Autodesk Fusion 360 part; units mm, degrees
note: some values were not read from the file. Chosen so that the rebuilt part matches the saved one: which face or edge a step refers to. Set by a fixed rule: which sketch regions a step uses; the direction of a hole.
(part 3 of 4)
sketch "Sketch120" plane through (0, -75, 0) normal (0, 1, 0) x (-1, 0, 0)
  line L0 (-100, 0) -> (-100, -5)
  line L1 (-100, -5) -> (-90, -5)
  line L2 (-90, -5) -> (-90, 3.5)
  line L3 (-90, 3.5) -> (-100, 3.5)
  line L4 (-100, 3.5) -> (-100, 50)
  line L5 (-100, 50) -> (-162.3, 50)
  line L6 (-162.3, 50) -> (-162.3, 3.5)
  line L7 (-162.3, 3.5) -> (-172.3, 3.5)
  line L8 (-172.3, 3.5) -> (-172.3, -5)
  line L9 (-172.3, -5) -> (-162.3, -5)
  line L10 (-162.3, -5) -> (-162.3, 0)
  line L11 (-162.3, 0) -> (-100, 0)
  line L12 (-162.3, 45) -> (-152.3, 45)
  line L13 (-152.3, 45) -> (-152.3, 42)
  line L14 (-152.3, 42) -> (-162.3, 42)
  line L15 (-162.3, 42) -> (-162.3, 45)
  line L16 (-100, 45) -> (-110, 45)
  line L17 (-110, 45) -> (-110, 42)
  line L18 (-110, 42) -> (-100, 42)
  line L19 (-100, 42) -> (-100, 45)
  line L20 (-162.3, 50) -> (-100, 50)
  dimension "d903" = 10
  dimension "d904" = 3
  dimension "d905" = 5
  dimension "d906" = 10
  dimension "d907" = 3
  dimension "d908" = 5
  constraint horizontal L12
  constraint vertical L13
  constraint horizontal L14
  constraint vertical L15
  constraint coincident L6 L12.start
  constraint horizontal L16
  constraint vertical L17
  constraint horizontal L18
  constraint vertical L19
  constraint coincident L4 L16.start
  measures "d903" distance of L12.start L12.end
  measures "d904" distance of L12.start L14.end
  measures "d905" distance of L5 L12
  measures "d906" distance of L16.start L16.end
  measures "d907" distance of L16.start L18.end
  measures "d908" distance of L16 L20
extrude "Extrude160" cut sketch "Sketch120" against normal blind 10 contours L4 L16 L17 L18 L19 | L6 L12 L13 L14 L15 bodies 7
extrude "Extrude161" add sketch "Sketch119" along normal blind 5 contours L4 L10 L14 L15 L16 L17 bodies 7
sketch "Sketch121" plane through (0, 0, 0) normal (0, 0, 1) x (1, 0, 0)
  line L0 (90, -100) -> (172.3, -100)
  line L1 (172.3, -100) -> (172.3, -145)
  line L2 (172.3, -145) -> (90, -145)
  line L3 (90, -145) -> (90, -100)
  line L4 (100, -100) -> (110, -100)
  line L5 (110, -100) -> (110, -110)
  line L6 (110, -110) -> (100, -110)
  line L7 (100, -110) -> (100, -100)
  line L8 (100, -145) -> (110, -145)
  line L9 (110, -145) -> (110, -135)
  line L10 (110, -135) -> (100, -135)
  line L11 (100, -135) -> (100, -145)
  line L12 (152.3, -100) -> (162.3, -100)
  line L13 (162.3, -100) -> (162.3, -110)
  line L14 (162.3, -110) -> (152.3, -110)
  line L15 (152.3, -110) -> (152.3, -100)
  line L16 (152.3, -145) -> (162.3, -145)
  line L17 (162.3, -145) -> (162.3, -135)
  line L18 (162.3, -135) -> (152.3, -135)
  line L19 (152.3, -135) -> (152.3, -145)
  circle A0 centre (105, -105) radius 2.5
  circle A1 centre (105, -140) radius 2.5
  circle A2 centre (157.3, -140) radius 2.5
  circle A3 centre (157.3, -105) radius 2.5
  line L20 (110, -100) -> (152.3, -100)
  line L21 (152.3, -100) -> (152.3, -110)
  line L22 (152.3, -110) -> (110, -110)
  line L23 (110, -110) -> (110, -100)
  line L24 (110, -135) -> (152.3, -135)
  line L25 (152.3, -135) -> (152.3, -145)
  line L26 (152.3, -145) -> (110, -145)
  line L27 (110, -145) -> (110, -135)
  circle A4 centre (131.15, -122.5) radius 8.5
  line L28 (172.3, -100) -> (90, -100)
  line L29 (90, -100) -> (90, -97)
  line L30 (90, -97) -> (172.3, -97)
  line L31 (172.3, -97) -> (172.3, -100)
  line L32 (90, -145) -> (172.3, -145)
  line L33 (172.3, -145) -> (172.3, -148)
  line L34 (172.3, -148) -> (90, -148)
  line L35 (90, -148) -> (90, -145)
  circle A5 centre (152.3, -110) radius 1
  circle A6 centre (152.3, -100) radius 1
  circle A7 centre (110, -110) radius 1
  circle A8 centre (110, -100) radius 1
  circle A9 centre (110, -135) radius 1
  circle A10 centre (110, -145) radius 1
  circle A11 centre (152.3, -145) radius 1
  circle A12 centre (152.3, -135) radius 1
  dimension "d913" = 82.3
  dimension "d914" = 45
  dimension "d915" = 10
  dimension "d916" = 10
  dimension "d917" = 10
  dimension "d918" = 10
  dimension "d919" = 10
  dimension "d920" = 5
  dimension "d921" = 5
  dimension "d922" = 5
  dimension "d923" = 5
  dimension "d930" = 17
  dimension "d1117" = 3
  dimension "d1118" = 3
  dimension "d1119" = 2
  dimension "d1120" = 2
  dimension "d1121" = 2
  dimension "d1122" = 2
  dimension "d1123" = 2
  dimension "d1124" = 2
  dimension "d1125" = 2
  dimension "d1126" = 2
  constraint horizontal L0
  constraint vertical L1
  constraint horizontal L2
  constraint vertical L3
  constraint horizontal L4
  constraint vertical L5
  constraint horizontal L6
  constraint vertical L7
  constraint coincident L0 L4.start
  constraint horizontal L8
  constraint vertical L9
  constraint horizontal L10
  constraint vertical L11
  constraint coincident L2 L8.start
  constraint horizontal L12
  constraint vertical L13
  constraint horizontal L14
  constraint vertical L15
  constraint coincident L0 L12.start
  constraint horizontal L16
  constraint vertical L17
  constraint horizontal L18
  constraint vertical L19
  constraint coincident L2 L16.start
  constraint horizontal L20
  constraint vertical L21
  constraint horizontal L22
  constraint vertical L23
  constraint horizontal L24
  constraint vertical L25
  constraint horizontal L26
  constraint vertical L27
  constraint horizontal L28
  constraint vertical L29
  constraint horizontal L30
  constraint vertical L31
  constraint horizontal L32
  constraint vertical L33
  constraint horizontal L34
  constraint vertical L35
  constraint coincident L14.end L15.start
  constraint coincident L12.start L15.end
  constraint coincident L5.end L6.start
  constraint coincident L4.end L5.start
  constraint coincident L9.end L10.start
  constraint coincident L8.end L9.start
  constraint coincident L16.start L19.end
  constraint coincident L18.end L19.start
  measures "d913" distance of L0.start L0.end
  measures "d914" distance of L0.start L2.end
  measures "d915" distance of L12.start L12.end
  measures "d916" distance of L16.start L16.end
  measures "d917" distance of L16.start L18.end
  measures "d918" distance of L1 L13
  measures "d919" distance of L1 L17
  measures "d920" diameter of A0
  measures "d921" diameter of A1
  measures "d922" diameter of A2
  measures "d923" diameter of A3
  measures "d930" diameter of A4
  measures "d1117" distance of L2.end L34.end
  measures "d1118" distance of L0.end L30.end
  measures "d1119" diameter of A5
  measures "d1120" diameter of A6
  measures "d1121" diameter of A7
  measures "d1122" diameter of A8
  measures "d1123" diameter of A9
  measures "d1124" diameter of A10
  measures "d1125" diameter of A11
  measures "d1126" diameter of A12
extrude "Extrude162" add sketch "Sketch121" along normal blind 10 separate body contours L0 L4 L12 L20 L28 L29 L30 L31 A6 A8 | L0 L1 L2 L3 L6 L7 L10 L11 L13 L14 L17 L18 L22 L24 L28 L32 A5 A7 A9 A12 | L0 L4 L5 L6 L7 L23 L28 A7 A8 | L2 L8 L16 L26 L32 L33 L34 L35 A10 A11 | L2 L8 L9 L10 L11 L27 L32 A9 A10 | L0 L12 L13 L14 L15 L21 L28 A5 A6 | L2 L16 L17 L18 L19 L25 L32 A11 A12 | A4 makes body 9
extrude "Extrude163" add sketch "Sketch121" along normal blind 5 contours L0 L4 L20 L28 A8 | L0 L4 L5 L23 L28 A8 | L0 L5 L20 L23 L28 A8 | L0 L5 L15 L20 L21 L22 L23 L28 A5 A6 A7 A8 | L5 L6 L23 A7 | L6 L22 A7 | L2 L8 L9 L27 L32 A10 | L2 L8 L26 L32 A10 | L0 L12 L20 L28 A6 | L0 L15 L20 L21 L28 A6 | L5 L22 L23 A7 | L2 L9 L26 L27 L32 A10 | L2 L9 L19 L24 L25 L26 L27 L32 A9 A10 A11 A12 | L10 L24 A9 | L9 L10 L27 A9 | L0 L12 L15 L21 L28 A6 | L15 L21 L22 A5 | L14 L22 A5 | L9 L24 L27 A9 | L2 L19 L25 L26 L32 A11 | L2 L16 L26 L32 A11 | L14 L15 L21 A5 | L2 L16 L19 L25 L32 A11 | L18 L24 A12 | L19 L24 L25 A12 | L18 L19 L25 A12 bodies 9
extrude "Extrude164" add sketch "Sketch121" along normal blind 5 contours L0 L4 L12 L20 L28 L29 L30 L31 A6 A8 | L0 L4 L5 L6 L7 L23 L28 A7 A8 | L2 L8 L16 L26 L32 L33 L34 L35 A10 A11 | L2 L8 L9 L10 L11 L27 L32 A9 A10 | L5 L6 L23 A7 | L9 L10 L27 A9 | L0 L12 L13 L14 L15 L21 L28 A5 A6 | L2 L16 L17 L18 L19 L25 L32 A11 A12 bodies 9
sketch "Sketch122" plane through (0, 0, 10) normal (0, 0, 1) x (-1, 0, 0)
  line L0 (-172.3, 148) -> (-172.3, 97)
  line L1 (-90, 97) -> (-90, 148)
  circle A0 centre (-131.15, 122.5) radius 8.5
  arc A1 (-111, 135) -> (-110, 136) centre (-110, 135) ccw
  arc A2 (-152.3, 136) -> (-151.3, 135) centre (-152.3, 135) ccw
  arc A3 (-151.3, 110) -> (-152.3, 109) centre (-152.3, 110) ccw
  arc A4 (-110, 109) -> (-111, 110) centre (-110, 110) ccw
  line L2 (-151.3, 110) -> (-111, 110)
  line L3 (-111, 135) -> (-151.3, 135)
  arc A5 (-151.3, 145) -> (-152.3, 144) centre (-152.3, 145) ccw
  line L4 (-151.3, 145) -> (-111, 145)
  arc A6 (-110, 144) -> (-111, 145) centre (-110, 145) ccw
  arc A7 (-111, 100) -> (-110, 101) centre (-110, 100) ccw
  line L5 (-111, 100) -> (-151.3, 100)
  arc A8 (-152.3, 101) -> (-151.3, 100) centre (-152.3, 100) ccw
  line L6 (-90, 148) -> (-172.3, 148)
  line L7 (-172.3, 97) -> (-90, 97)
  circle A9 centre (-105, 105) radius 2.5
  line L8 (-152.3, 101) -> (-152.3, 109)
  line L9 (-110, 109) -> (-110, 101)
  circle A10 centre (-157.3, 140) radius 2.5
  circle A11 centre (-157.3, 105) radius 2.5
  line L10 (-110, 144) -> (-110, 136)
  line L11 (-152.3, 136) -> (-152.3, 144)
  circle A12 centre (-105, 140) radius 2.5
  dimension "d931" = 17
  measures "d931" diameter of A0
hole "Hole32" at (131.15, -122.5, 10) direction (0, 0, -1) diameter 16 depth 10 tip angle 180 countersink diameter 17 countersink angle 30 bodies 9
sketch "Sketch123" plane through (0, 0, 0) normal (0, 0, 1) x (1, 0, 0)
  line L0 (85, -150) -> (167.3, -150)
  line L1 (167.3, -150) -> (167.3, -175)
  line L2 (167.3, -175) -> (85, -175)
  line L3 (85, -175) -> (85, -150)
  line L4 (105, -150) -> (110, -150)
  line L5 (110, -150) -> (110, -155)
  line L6 (110, -155) -> (105, -155)
  line L7 (105, -155) -> (105, -150)
  line L8 (142.3, -150) -> (147.3, -150)
  line L9 (147.3, -150) -> (147.3, -155)
  line L10 (147.3, -155) -> (142.3, -155)
  line L11 (142.3, -155) -> (142.3, -150)
  line L12 (147.3, -175) -> (142.3, -175)
  line L13 (142.3, -175) -> (142.3, -170)
  line L14 (142.3, -170) -> (147.3, -170)
  line L15 (147.3, -170) -> (147.3, -175)
  line L16 (105, -175) -> (110, -175)
  line L17 (110, -175) -> (110, -170)
  line L18 (110, -170) -> (105, -170)
  line L19 (105, -170) -> (105, -175)
  line L20 (147.3, -155) -> (148.3, -155)
  line L21 (148.3, -155) -> (147.3, -150)
  line L22 (142.3, -155) -> (141.3, -155)
  line L23 (141.3, -155) -> (142.3, -150)
  line L24 (110, -155) -> (111, -155)
  line L25 (111, -155) -> (110, -150)
  line L26 (105, -155) -> (104, -155)
  line L27 (104, -155) -> (105, -150)
  line L28 (105, -170) -> (104, -170)
  line L29 (104, -170) -> (105, -175)
  line L30 (110, -170) -> (111, -170)
  line L31 (111, -170) -> (110, -175)
  line L32 (142.3, -170) -> (141.3, -170)
  line L33 (141.3, -170) -> (142.3, -175)
  line L34 (147.3, -170) -> (148.3, -170)
  line L35 (148.3, -170) -> (147.3, -175)
  circle A0 centre (111, -170) radius 1
  circle A1 centre (104, -170) radius 1
  circle A2 centre (105, -175) radius 1
  circle A3 centre (110, -175) radius 1
  circle A4 centre (142.3, -175) radius 1
  circle A5 centre (147.3, -175) radius 1
  circle A6 centre (148.3, -170) radius 1
  circle A7 centre (141.3, -170) radius 1
  circle A8 centre (148.3, -155) radius 1
  circle A9 centre (141.3, -155) radius 1
  circle A10 centre (111, -155) radius 1
  circle A11 centre (104, -155) radius 1
  line L36 (167.3, -150) -> (177.3, -150)
  line L37 (177.3, -150) -> (177.3, -175)
  line L38 (177.3, -175) -> (167.3, -175)
  line L39 (167.3, -175) -> (167.3, -150)
  line L40 (85, -150) -> (75, -150)
  line L41 (75, -150) -> (75, -175)
  line L42 (75, -175) -> (85, -175)
  line L43 (85, -175) -> (85, -150)
  line L44 (75, -150) -> (82.5, -150)
  line L45 (82.5, -150) -> (82.5, -175)
  line L46 (82.5, -175) -> (75, -175)
  line L47 (75, -175) -> (75, -150)
  line L48 (177.3, -150) -> (169.8, -150)
  line L49 (169.8, -150) -> (169.8, -175)
  line L50 (169.8, -175) -> (177.3, -175)
  line L51 (177.3, -175) -> (177.3, -150)
  circle A12 centre (142.3, -150) radius 1
  circle A13 centre (147.3, -150) radius 1
  circle A14 centre (110, -150) radius 1
  circle A15 centre (105, -150) radius 1
  dimension "d937" = 82.3
  dimension "d938" = 25
  dimension "d939" = 32.3
  dimension "d940" = 20
  dimension "d941" = 20
  dimension "d942" = 32.3
  dimension "d943" = 1
  dimension "d944" = 1
  dimension "d945" = 1
  dimension "d946" = 1
  dimension "d947" = 1
  dimension "d948" = 1
  dimension "d949" = 1
  dimension "d950" = 1
  dimension "d951" = 2
  dimension "d952" = 2
  dimension "d953" = 2
  dimension "d954" = 2
  dimension "d955" = 2
  dimension "d956" = 2
  dimension "d957" = 2
  dimension "d958" = 2
  dimension "d959" = 2
  dimension "d960" = 2
  dimension "d961" = 2
  dimension "d962" = 2
  dimension "d963" = 10
  dimension "d964" = 10
  dimension "d965" = 7.5
  dimension "d966" = 7.5
  dimension "d967" = 2
  dimension "d968" = 2
  dimension "d969" = 2
  dimension "d970" = 2
  constraint horizontal L0
  constraint vertical L1
  constraint horizontal L2
  constraint vertical L3
  constraint horizontal L4
  constraint vertical L5
  constraint horizontal L6
  constraint vertical L7
  constraint coincident L0 L4.start
  constraint horizontal L8
  constraint vertical L9
  constraint horizontal L10
  constraint vertical L11
  constraint coincident L0 L8.start
  constraint horizontal L12
  constraint vertical L13
  constraint horizontal L14
  constraint vertical L15
  constraint coincident L2 L12.start
  constraint horizontal L16
  constraint vertical L17
  constraint horizontal L18
  constraint vertical L19
  constraint coincident L2 L16.start
  constraint perpendicular L9 L20
  constraint perpendicular L11 L22
  constraint perpendicular L5 L24
  constraint perpendicular L7 L26
  constraint perpendicular L19 L28
  constraint perpendicular L17 L30
  constraint perpendicular L13 L32
  constraint perpendicular L15 L34
  constraint coincident L30.end L31.start
  constraint coincident L28.end L29.start
  constraint coincident L16.start L19.end
  constraint coincident L16.end L17.start
  constraint coincident L12.end L13.start
  constraint coincident L12.start L15.end
  constraint coincident L34.end L35.start
  constraint coincident L32.end L33.start
  constraint coincident L20.end L21.start
  constraint coincident L22.end L23.start
  constraint coincident L24.end L25.start
  constraint coincident L26.end L27.start
  constraint horizontal L36
  constraint vertical L37
  constraint horizontal L38
  constraint vertical L39
  constraint horizontal L40
  constraint vertical L41
  constraint horizontal L42
  constraint vertical L43
  constraint horizontal L44
  constraint vertical L45
  constraint horizontal L46
  constraint vertical L47
  constraint horizontal L48
  constraint vertical L49
  constraint horizontal L50
  constraint vertical L51
  constraint coincident L8.start L11.end
  constraint coincident L8.end L9.start
  constraint coincident L4.end L5.start
  constraint coincident L4.start L7.end
  measures "d937" distance of L0.start L0.end
  measures "d938" distance of L0.start L2.end
  measures "d939" distance of L5 L11
  measures "d940" distance of L3 L7
  measures "d941" distance of L3 L19
  measures "d942" distance of L13 L17
  measures "d943" distance of L9.end L20.end
  measures "d944" distance of L10.end L22.end
  measures "d945" distance of L5.end L24.end
  measures "d946" distance of L6.end L26.end
  measures "d947" distance of L18.end L28.end
  measures "d948" distance of L17.end L30.end
  measures "d949" distance of L13.end L32.end
  measures "d950" distance of L14.end L34.end
  measures "d951" diameter of A0
  measures "d952" diameter of A1
  measures "d953" diameter of A2
  measures "d954" diameter of A3
  measures "d955" diameter of A4
  measures "d956" diameter of A5
  measures "d957" diameter of A6
  measures "d958" diameter of A7
  measures "d959" diameter of A8
  measures "d960" diameter of A9
  measures "d961" diameter of A10
  measures "d962" diameter of A11
  measures "d963" distance of L0.end L36.end
  measures "d964" distance of L0.start L40.end
  measures "d965" distance of L40.end L44.end
  measures "d966" distance of L36.end L48.end
  measures "d967" diameter of A12
  measures "d968" diameter of A13
  measures "d969" diameter of A14
  measures "d970" diameter of A15
extrude "Extrude165" add sketch "Sketch123" along normal blind 15 separate body contours L0 L1 L2 L3 L6 L10 L14 L18 L21 L23 L25 L27 L29 L31 L33 L35 A0 A1 A2 A3 A4 A5 A6 A7 A8 A9 A10 A11 L39 L43 A12 A13 A14 A15 | L3 L40 L42 L43 L45 | L1 L36 L38 L39 L49 makes body 10
extrude "Extrude166" add sketch "Sketch123" along normal blind 67 contours L40 L41 L42 L44 L45 L46 L47 | L36 L37 L38 L48 L49 L50 L51 bodies 10
sketch "Sketch124" plane through (0, 0, 15) normal (0, 0, 1) x (-1, 0, 0)
  line L0 (-82.5, 150) -> (-82.5, 175)
  line L1 (-82.5, 175) -> (-85, 175)
  line L2 (-85, 175) -> (-104, 175)
  arc A0 (-104.8039, 174.0194) -> (-104, 175) centre (-105, 175) ccw
  line L3 (-104.8039, 174.0194) -> (-104.1961, 170.9806)
  arc A1 (-105, 170) -> (-104.1961, 170.9806) centre (-104, 170) ccw
  line L4 (-105, 170) -> (-110, 170)
  arc A2 (-110.8039, 170.9806) -> (-110, 170) centre (-111, 170) ccw
  line L5 (-110.8039, 170.9806) -> (-110.1961, 174.0194)
  arc A3 (-111, 175) -> (-110.1961, 174.0194) centre (-110, 175) ccw
  line L6 (-111, 175) -> (-141.3, 175)
  arc A4 (-142.1039, 174.0194) -> (-141.3, 175) centre (-142.3, 175) ccw
  line L7 (-142.1039, 174.0194) -> (-141.4961, 170.9806)
  arc A5 (-142.3, 170) -> (-141.4961, 170.9806) centre (-141.3, 170) ccw
  line L8 (-142.3, 170) -> (-147.3, 170)
  arc A6 (-148.1039, 170.9806) -> (-147.3, 170) centre (-148.3, 170) ccw
  line L9 (-148.1039, 170.9806) -> (-147.4961, 174.0194)
  arc A7 (-148.3, 175) -> (-147.4961, 174.0194) centre (-147.3, 175) ccw
  line L10 (-148.3, 175) -> (-167.3, 175)
  line L11 (-167.3, 175) -> (-169.8, 175)
  line L12 (-169.8, 175) -> (-169.8, 150)
  line L13 (-169.8, 150) -> (-148.3, 150)
  arc A8 (-147.4961, 150.9806) -> (-148.3, 150) centre (-147.3, 150) ccw
  line L14 (-147.4961, 150.9806) -> (-148.1039, 154.0194)
  arc A9 (-147.3, 155) -> (-148.1039, 154.0194) centre (-148.3, 155) ccw
  line L15 (-147.3, 155) -> (-142.3, 155)
  arc A10 (-141.4961, 154.0194) -> (-142.3, 155) centre (-141.3, 155) ccw
  line L16 (-141.4961, 154.0194) -> (-142.1039, 150.9806)
  arc A11 (-141.3, 150) -> (-142.1039, 150.9806) centre (-142.3, 150) ccw
  line L17 (-141.3, 150) -> (-111, 150)
  arc A12 (-110.1961, 150.9806) -> (-111, 150) centre (-110, 150) ccw
  line L18 (-110.1961, 150.9806) -> (-110.8039, 154.0194)
  arc A13 (-110, 155) -> (-110.8039, 154.0194) centre (-111, 155) ccw
  line L19 (-110, 155) -> (-105, 155)
  arc A14 (-104.1961, 154.0194) -> (-105, 155) centre (-104, 155) ccw
  line L20 (-104.1961, 154.0194) -> (-104.8039, 150.9806)
  arc A15 (-104, 150) -> (-104.8039, 150.9806) centre (-105, 150) ccw
  line L21 (-104, 150) -> (-82.5, 150)
  circle A16 centre (-126.15, 162.5) radius 7.5
  dimension "d975" = 15
  measures "d975" diameter of A16
extrude "Extrude175" add sketch "Sketch123" against normal blind 7.5 contours L0 L1 L2 L3 L6 L10 L14 L18 L21 L23 L25 L27 L29 L31 L33 L35 A0 A1 A2 A3 A4 A5 A6 A7 A8 A9 A10 A11 L39 L43 A12 A13 A14 A15 | L3 L40 L42 L43 L45 | L40 L41 L42 L44 L45 L46 L47 | L1 L36 L38 L39 L49 | L36 L37 L38 L48 L49 L50 L51 bodies 10
extrude "Extrude176" add 1 faces at (90.2093, -160.1631, 15) along direction (0, 0, 1) blind 7.5 on bodies 10 bodies 10
sketch "Sketch134" plane through (0, 0, 22.5) normal (0, 0, 1) x (-1, 0, 0)
  line L0 (-82.5, 150) -> (-82.5, 175)
  line L1 (-82.5, 175) -> (-85, 175)
  line L2 (-85, 175) -> (-104, 175)
  arc A0 (-104.8039, 174.0194) -> (-104, 175) centre (-105, 175) ccw
  line L3 (-104.8039, 174.0194) -> (-104.1961, 170.9806)
  arc A1 (-105, 170) -> (-104.1961, 170.9806) centre (-104, 170) ccw
  line L4 (-105, 170) -> (-110, 170)
  arc A2 (-110.8039, 170.9806) -> (-110, 170) centre (-111, 170) ccw
  line L5 (-110.8039, 170.9806) -> (-110.1961, 174.0194)
  arc A3 (-111, 175) -> (-110.1961, 174.0194) centre (-110, 175) ccw
  line L6 (-111, 175) -> (-141.3, 175)
  arc A4 (-142.1039, 174.0194) -> (-141.3, 175) centre (-142.3, 175) ccw
  line L7 (-142.1039, 174.0194) -> (-141.4961, 170.9806)
  arc A5 (-142.3, 170) -> (-141.4961, 170.9806) centre (-141.3, 170) ccw
  line L8 (-142.3, 170) -> (-147.3, 170)
  arc A6 (-148.1039, 170.9806) -> (-147.3, 170) centre (-148.3, 170) ccw
  line L9 (-148.1039, 170.9806) -> (-147.4961, 174.0194)
  arc A7 (-148.3, 175) -> (-147.4961, 174.0194) centre (-147.3, 175) ccw
  line L10 (-148.3, 175) -> (-167.3, 175)
  line L11 (-167.3, 175) -> (-169.8, 175)
  line L12 (-169.8, 175) -> (-169.8, 150)
  line L13 (-169.8, 150) -> (-148.3, 150)
  arc A8 (-147.4961, 150.9806) -> (-148.3, 150) centre (-147.3, 150) ccw
  line L14 (-147.4961, 150.9806) -> (-148.1039, 154.0194)
  arc A9 (-147.3, 155) -> (-148.1039, 154.0194) centre (-148.3, 155) ccw
  line L15 (-147.3, 155) -> (-142.3, 155)
  arc A10 (-141.4961, 154.0194) -> (-142.3, 155) centre (-141.3, 155) ccw
  line L16 (-141.4961, 154.0194) -> (-142.1039, 150.9806)
  arc A11 (-141.3, 150) -> (-142.1039, 150.9806) centre (-142.3, 150) ccw
  line L17 (-141.3, 150) -> (-111, 150)
  arc A12 (-110.1961, 150.9806) -> (-111, 150) centre (-110, 150) ccw
  line L18 (-110.1961, 150.9806) -> (-110.8039, 154.0194)
  arc A13 (-110, 155) -> (-110.8039, 154.0194) centre (-111, 155) ccw
  line L19 (-110, 155) -> (-105, 155)
  arc A14 (-104.1961, 154.0194) -> (-105, 155) centre (-104, 155) ccw
  line L20 (-104.1961, 154.0194) -> (-104.8039, 150.9806)
  arc A15 (-104, 150) -> (-104.8039, 150.9806) centre (-105, 150) ccw
  line L21 (-104, 150) -> (-82.5, 150)
  circle A16 centre (-126.15, 162.5) radius 7.5
  dimension "d1043" = 15
  measures "d1043" diameter of A16
sketch "Sketch125" plane through (177.3, 0, 0) normal (1, 0, 0) x (0, 1, 0)
  line L0 (-150, -7.5) -> (-150, 67)
  line L1 (-150, 67) -> (-175, 67)
  line L2 (-150, 67) -> (-175, 67)
  line L3 (-175, 67) -> (-175, 57)
  line L4 (-175, 57) -> (-150, 57)
  line L5 (-150, 57) -> (-150, 67)
  line L6 (-175, 67) -> (-175, 0)
  line L7 (-175, -7.5) -> (-150, -7.5)
  line L8 (-175, 0) -> (-175, -7.5)
  dimension "d981" = 10
  constraint horizontal L2
  constraint vertical L3
  constraint horizontal L4
  constraint vertical L5
  constraint coincident L0.end L1.start
  measures "d981" distance of L0.end L4.end
sketch "Sketch126" plane through (75, 0, 0) normal (-1, 0, 0) x (0, -1, 0)
  line L0 (175, -7.5) -> (175, 67)
  line L1 (175, 67) -> (150, 67)
  line L2 (150, 67) -> (150, -7.5)
  line L3 (150, 67) -> (175, 67)
  line L4 (175, 67) -> (175, 57)
  line L5 (175, 57) -> (150, 57)
  line L6 (150, 57) -> (150, 67)
  line L7 (150, -7.5) -> (175, -7.5)
  dimension "d992" = 10
  constraint horizontal L3
  constraint vertical L4
  constraint horizontal L5
  constraint vertical L6
  constraint coincident L0 L4.end
  constraint coincident L1.end L2.start
  measures "d992" distance of L0.end L4.end
extrude "Extrude167" add sketch "Sketch126" along normal blind 10 contours L0 L1 L2 L3 L4 L5 L6 bodies 10
extrude "Extrude168" add sketch "Sketch125" along normal blind 10 contours L0 L1 L2 L3 L4 L5 L6 bodies 10
sketch "Sketch127" plane through (0, -175, 0) normal (0, -1, 0) x (1, 0, 0)
  line L0 (82.5, 22.5) -> (82.5, 67)
  line L1 (82.5, 67) -> (65, 67)
  line L2 (65, 67) -> (65, 57)
  line L3 (65, 57) -> (75, 57)
  line L4 (75, 57) -> (75, -7.5)
  circle A0 centre (75, 59.5) radius 7.5
  line L5 (75, 57) -> (65, 57)
  line L6 (65, 57) -> (65, 67)
  line L7 (65, 67) -> (75, 67)
  line L8 (75, 67) -> (75, 57)
  line L9 (75, -7.5) -> (85, -7.5)
  line L10 (85, -7.5) -> (104, -7.5)
  line L11 (104, 0) -> (104, 15)
  line L12 (104, 15) -> (104, 22.5)
  line L13 (104, 22.5) -> (85, 22.5)
  line L14 (85, 22.5) -> (82.5, 22.5)
  line L15 (104, -7.5) -> (104, 0)
  constraint tangent L0 A0
  constraint tangent L1 A0
  constraint horizontal L5
  constraint vertical L6
  constraint horizontal L7
  constraint vertical L8
  constraint coincident L1.end L2.start
  constraint coincident L3.end L4.start
extrude "Extrude169" cut sketch "Sketch127" against normal blind 30.349 contours L0 L1 A0 bodies 10
sketch "Sketch128" plane through (0, -175, 0) normal (0, -1, 0) x (1, 0, 0)
  line L0 (177.3, 57) -> (187.3, 57)
  line L1 (187.3, 57) -> (187.3, 67)
  line L2 (187.3, 67) -> (169.8, 67)
  line L3 (169.8, 67) -> (169.8, 22.5)
  line L4 (148.3, 22.5) -> (148.3, -7.5)
  circle A0 centre (177.3, 59.5) radius 7.5
  line L5 (187.3, 57) -> (177.3, 57)
  line L6 (177.3, 57) -> (177.3, 67)
  line L7 (177.3, 67) -> (187.3, 67)
  line L8 (187.3, 67) -> (187.3, 57)
  line L9 (148.3, -7.5) -> (167.3, -7.5)
  line L10 (167.3, -7.5) -> (177.3, -7.5)
  line L11 (177.3, -7.5) -> (177.3, 0)
  line L12 (169.8, 22.5) -> (167.3, 22.5)
  line L13 (167.3, 22.5) -> (148.3, 22.5)
  line L14 (177.3, 0) -> (177.3, 57)
  constraint tangent L3 A0
  constraint tangent L2 A0
  constraint horizontal L5
  constraint vertical L6
  constraint horizontal L7
  constraint vertical L8
  constraint coincident A0 L6.end
  constraint coincident L0.end L1.start
extrude "Extrude170" cut sketch "Sketch128" against normal blind 30.066 contours L2 L3 A0 bodies 10
extrude "Extrude171" add sketch "Sketch128" sketch "Sketch127" along normal blind 41 contours L0 A0 L5 L6 | L0 L1 L2 A0 L5 L7 L8 of sketch 2 contours L1 L2 L3 A0 L5 L6 L7 | L3 A0 L5 L8 bodies 10
sketch "Sketch129" plane through (177.3, 0, 0) normal (-1, 0, 0) x (0, -1, 0)
  line L0 (175, 67) -> (175, 57)
  line L1 (175, 57) -> (216, 57)
  line L2 (216, 57) -> (216, 67)
  line L3 (216, 67) -> (175, 67)
  line L4 (216, 67) -> (186, 67)
  line L5 (186, 67) -> (186, 57)
  line L6 (186, 57) -> (216, 57)
  line L7 (216, 57) -> (216, 67)
  dimension "d993" = 30
  constraint horizontal L4
  constraint vertical L5
  constraint horizontal L6
  constraint vertical L7
  constraint coincident L2.end L3.start
  measures "d993" distance of L2.end L4.end
extrude "Extrude172" add sketch "Sketch129" along normal blind 103.7 contours L1 L2 L3 L4 L5 L6 L7 bodies 10
sketch "Sketch130" plane through (0, 0, 67) normal (0, 0, 1) x (-1, 0, 0)
  line L0 (-73.6, 216) -> (-75, 216)
  line L1 (-75, 216) -> (-187.3, 216)
  line L2 (-187.3, 216) -> (-187.3, 175)
  line L3 (-187.3, 175) -> (-187.3, 150)
  line L4 (-187.3, 150) -> (-177.3, 150)
  line L5 (-177.3, 150) -> (-177.3, 175)
  line L6 (-177.3, 175) -> (-177.3, 186)
  line L7 (-177.3, 186) -> (-75, 186)
  line L8 (-75, 186) -> (-75, 175)
  line L9 (-75, 175) -> (-75, 150)
  line L10 (-75, 150) -> (-65, 150)
  line L11 (-65, 150) -> (-65, 216)
  line L12 (-65, 216) -> (-73.6, 216)
  circle A0 centre (-90, 211) radius 1.5
  circle A1 centre (-162, 211) radius 1.5
  circle A2 centre (-152, 211) radius 1.5
  circle A3 centre (-80, 211) radius 1.5
  circle A4 centre (-172, 211) radius 1.5
  circle A5 centre (-100, 211) radius 1.5
  dimension "d996" = 3
  dimension "d997" = 3
  dimension "d998" = 25
  dimension "d999" = 25
  dimension "d1000" = 72
  dimension "d1001" = 25
  dimension "d1002" = 3
  dimension "d1003" = 3
  dimension "d1004" = 72
  dimension "d1005" = 25
  dimension "d1006" = 25
  dimension "d1007" = 15
  dimension "d1113" = 3
  dimension "d1114" = 10
  dimension "d1115" = 3
  dimension "d1116" = 72
  measures "d996" diameter of A0
  measures "d997" diameter of A1
  measures "d998" distance of L7 A0.centre
  measures "d999" distance of L7 A1.centre
  measures "d1000" distance of A0.centre A1.centre
  measures "d1001" distance of L11 A0.centre
  measures "d1002" diameter of A2
  measures "d1003" diameter of A3
  measures "d1004" distance of A2.centre A3.centre
  measures "d1005" distance of L7 A3.centre
  measures "d1006" distance of L7 A2.centre
  measures "d1007" distance of L11 A3.centre
  measures "d1113" diameter of A4
  measures "d1114" distance of A1.centre A4.centre
  measures "d1115" diameter of A5
  measures "d1116" distance of A4.centre A5.centre
hole "Hole34" at (162, -211, 67) at (152, -211, 67) at (90, -211, 67) at (80, -211, 67) at (100, -211, 67) at (172, -211, 67) direction (0, 0, -1) diameter 3 depth 10 tip angle 180 counterbore diameter 7 counterbore depth 3 bodies 10
sketch "Sketch132" plane through (0, 0, 0) normal (0, 0, 1) x (1, 0, 0)
  line L0 (-150, -190) -> (-70, -190)
  line L1 (-70, -190) -> (-70, -215)
  line L2 (-70, -215) -> (-150, -215)
  line L3 (-150, -215) -> (-150, -190)
  circle A0 centre (-145, -210) radius 1.5
  circle A1 centre (-73, -210) radius 1.5
  line L4 (-135, -197.5) -> (-120, -197.5)
  line L5 (-120, -197.5) -> (-120, -207.5)
  line L6 (-120, -207.5) -> (-135, -207.5)
  line L7 (-135, -207.5) -> (-135, -197.5)
  dimension "d1017" = 80
  dimension "d1018" = 25
  dimension "d1019" = 3
  dimension "d1020" = 3
  dimension "d1021" = 72
  dimension "d1022" = 5
  dimension "d1023" = 5
  dimension "d1036" = 10
  dimension "d1037" = 15
  dimension "d1038" = 15
  dimension "d1049" = 7.5
  constraint horizontal L0
  constraint vertical L1
  constraint horizontal L2
  constraint vertical L3
  constraint horizontal L4
  constraint vertical L5
  constraint horizontal L6
  constraint vertical L7
  measures "d1017" distance of L0.start L0.end
  measures "d1018" distance of L0.start L2.end
  measures "d1019" diameter of A0
  measures "d1020" diameter of A1
  measures "d1021" distance of A0.centre A1.centre
  measures "d1022" distance of L3 A0.centre
  measures "d1023" distance of L2 A0.centre
  measures "d1036" distance of L4.start L6.end
  measures "d1037" distance of L5.end L6.end
  measures "d1038" distance of L3 L7
  measures "d1049" distance of L2 L6
sketch "Sketch133" plane through (-135, 0, 0) normal (-1, 0, 0) x (0, -1, 0)
  line L0 (207.5, 0) -> (207.5, 25)
  line L1 (207.5, 25) -> (197.5, 25)
  line L2 (197.5, 25) -> (197.5, 0)
  circle A0 centre (202.5, 20) radius 3
  line L3 (197.5, 0) -> (207.5, 0)
  dimension "d1028" = 6
  dimension "d1029" = 5
  measures "d1028" diameter of A0
  measures "d1029" distance of L0 A0.centre
sketch "Sketch135" plane through (0, 235, 0) normal (0, 1, 0) x (-1, 0, 0)
  line L0 (32.5135, 23) -> (32.5135, 0)
  line L1 (32.5135, 0) -> (77.5135, 0)
  line L2 (77.5135, 0) -> (77.5135, 23)
  line L3 (33.0135, 23) -> (38.0135, 23)
  line L4 (38.0135, 23) -> (38.0135, 7)
  line L5 (38.0135, 7) -> (33.0135, 7)
  line L6 (33.0135, 7) -> (33.0135, 23)
  circle A0 centre (55.0135, 12.75) radius 8.5
  line L7 (77.5135, 23) -> (32.5135, 23)
  line L8 (30.0135, 0) -> (80.0135, 0)
  dimension "d1050" = 5
  dimension "d1063" = 0.5
  dimension "d1088" = 7
  dimension "d1089" = 16
  constraint horizontal L3
  constraint vertical L4
  constraint horizontal L5
  constraint vertical L6
  measures "d1050" distance of L3.start L3.end
  measures "d1063" distance of L0 L6
  measures "d1088" distance of L5 L8
  measures "d1089" distance of L3.end L4.end
extrude "Extrude177" add sketch "Sketch135" along normal blind 76 contours L3 L4 L5 L6 L7 bodies 4
sketch "Sketch136" plane through (-38.0135, 0, 0) normal (-1, 0, 0) x (0, -1, 0)
  line L0 (-235, 23) -> (-311, 23)
  line L1 (-311, 23) -> (-311, 7)
  line L2 (-311, 7) -> (-235, 7)
  circle A0 centre (-308.8, 19) radius 1.5
  circle A1 centre (-308.8, 10) radius 1.5
  line L3 (-235, 7) -> (-235, 23)
  dimension "d1053" = 3
  dimension "d1054" = 3
  dimension "d1055" = 9
  dimension "d1058" = 3
  dimension "d1136" = 73.8
  dimension "d1137" = 73.8
  measures "d1053" diameter of A0
  measures "d1054" diameter of A1
  measures "d1055" vertical distance of A0.centre A1.centre
  measures "d1058" distance of L2 A1.centre
  measures "d1136" distance of A0.centre L3
  measures "d1137" distance of A1.centre L3
extrude "Extrude178" cut sketch "Sketch136" against normal blind 11.475 contours A0 | A1 bodies 4
sketch "Sketch137" plane through (0, 0, 0) normal (0, 0, 1) x (1, 0, 0)
  line L0 (-100, 200) -> (-105, 200)
  line L1 (-105, 200) -> (-105, 240)
  line L2 (-105, 240) -> (-100, 240)
  line L3 (-100, 240) -> (-100, 200)
  line L4 (-105, 200) -> (-147, 200)
  line L5 (-147, 200) -> (-147, 240)
  line L6 (-147, 240) -> (-105, 240)
  line L7 (-105, 240) -> (-105, 200)
  circle A0 centre (-142.8, 225.8) radius 1.5
  circle A1 centre (-142.8, 235) radius 1.5
  dimension "d1064" = 42
  dimension "d1065" = 3
  dimension "d1066" = 3
  dimension "d1067" = 9.2
  dimension "d1068" = 4.2
  dimension "d1079" = 40
  dimension "d1096" = 5
  constraint horizontal L0
  constraint vertical L1
  constraint horizontal L2
  constraint vertical L3
  constraint horizontal L4
  constraint vertical L5
  constraint horizontal L6
  constraint vertical L7
  measures "d1064" distance of L0.end L4.end
  measures "d1065" diameter of A0
  measures "d1066" diameter of A1
  measures "d1067" distance of A0.centre A1.centre
  measures "d1068" distance of L5 A0.centre
  measures "d1079" distance of L4.end L5.end
  measures "d1096" distance of L6 A1.centre
extrude "Extrude180" add sketch "Sketch137" along normal blind 15 separate body contours L0 L1 L2 L3 L7 makes body 11
extrude "Extrude181" add sketch "Sketch137" along normal blind 5 contours L1 L4 L5 L6 L7 bodies 11
sketch "Sketch138" plane through (-105, 0, 0) normal (-1, 0, 0) x (0, -1, 0)
  line L0 (-240, 5) -> (-200, 5)
  line L1 (-200, 5) -> (-200, 15)
  line L2 (-200, 15) -> (-240, 15)
  line L3 (-240, 15) -> (-240, 5)
  circle A0 centre (-235.5, 10.65) radius 1.5
  circle A1 centre (-204.5, 10.65) radius 1.5
  dimension "d1080" = 3
  dimension "d1081" = 3
  dimension "d1082" = 5.65
  dimension "d1083" = 5.65
  dimension "d1084" = 31
  dimension "d1085" = 4.5
  measures "d1080" diameter of A0
  measures "d1081" diameter of A1
  measures "d1082" distance of L0 A0.centre
  measures "d1083" distance of L0 A1.centre
  measures "d1084" distance of A0.centre A1.centre
  measures "d1085" distance of L3 A0.centre
extrude "Extrude182" cut sketch "Sketch138" against normal blind 9.531 contours A0 | A1 bodies 11
sketch "Sketch140" plane through (0, 0, 5) normal (0, 0, 1) x (-1, 0, 0)
  circle A0 centre (142.8, -225.8) radius 1.5
  circle A1 centre (142.8, -235) radius 1.5
  line L0 (105, -240) -> (147, -240)
  line L1 (147, -240) -> (147, -200)
  line L2 (147, -200) -> (105, -200)
  line L3 (105, -200) -> (105, -240)
  circle A2 centre (142.8, -225.8) radius 1.5
  circle A3 centre (142.8, -235) radius 1.5
  constraint concentric A0 A2
  constraint concentric A1 A3
hole "Hole38" at (-142.8, 235, 5) at (-142.8, 225.8, 5) direction (0, 0, -1) diameter 3 depth 7 tip angle 180 counterbore diameter 7 counterbore depth 3 bodies 11
extrude "Extrude183" add 1 faces at (90.2093, -160.1631, 22.5) along direction (0, 0, 1) blind 5 on bodies 10 bodies 10
extrude "Extrude184" add 1 faces at (87.6794, -160.0913, -7.5) along direction (0, 0, -1) blind 5 on bodies 10 bodies 10
sketch "Sketch141" plane through (0, 0, 27.5) normal (0, 0, 1) x (-1, 0, 0)
  line L0 (-82.5, 150) -> (-82.5, 175)
  line L1 (-82.5, 175) -> (-85, 175)
  line L2 (-85, 175) -> (-104, 175)
  arc A0 (-104.8039, 174.0194) -> (-104, 175) centre (-105, 175) ccw
  line L3 (-104.8039, 174.0194) -> (-104.1961, 170.9806)
  arc A1 (-105, 170) -> (-104.1961, 170.9806) centre (-104, 170) ccw
  line L4 (-105, 170) -> (-110, 170)
  arc A2 (-110.8039, 170.9806) -> (-110, 170) centre (-111, 170) ccw
  line L5 (-110.8039, 170.9806) -> (-110.1961, 174.0194)
  arc A3 (-111, 175) -> (-110.1961, 174.0194) centre (-110, 175) ccw
  line L6 (-111, 175) -> (-141.3, 175)
  arc A4 (-142.1039, 174.0194) -> (-141.3, 175) centre (-142.3, 175) ccw
  line L7 (-142.1039, 174.0194) -> (-141.4961, 170.9806)
  arc A5 (-142.3, 170) -> (-141.4961, 170.9806) centre (-141.3, 170) ccw
  line L8 (-142.3, 170) -> (-147.3, 170)
  arc A6 (-148.1039, 170.9806) -> (-147.3, 170) centre (-148.3, 170) ccw
  line L9 (-148.1039, 170.9806) -> (-147.4961, 174.0194)
  arc A7 (-148.3, 175) -> (-147.4961, 174.0194) centre (-147.3, 175) ccw
  line L10 (-148.3, 175) -> (-167.3, 175)
  line L11 (-167.3, 175) -> (-169.8, 175)
  line L12 (-169.8, 175) -> (-169.8, 150)
  line L13 (-169.8, 150) -> (-148.3, 150)
  arc A8 (-147.4961, 150.9806) -> (-148.3, 150) centre (-147.3, 150) ccw
  line L14 (-147.4961, 150.9806) -> (-148.1039, 154.0194)
  arc A9 (-147.3, 155) -> (-148.1039, 154.0194) centre (-148.3, 155) ccw
  line L15 (-147.3, 155) -> (-142.3, 155)
  arc A10 (-141.4961, 154.0194) -> (-142.3, 155) centre (-141.3, 155) ccw
  line L16 (-141.4961, 154.0194) -> (-142.1039, 150.9806)
  arc A11 (-141.3, 150) -> (-142.1039, 150.9806) centre (-142.3, 150) ccw
  line L17 (-141.3, 150) -> (-111, 150)
  arc A12 (-110.1961, 150.9806) -> (-111, 150) centre (-110, 150) ccw
  line L18 (-110.1961, 150.9806) -> (-110.8039, 154.0194)
  arc A13 (-110, 155) -> (-110.8039, 154.0194) centre (-111, 155) ccw
  line L19 (-110, 155) -> (-105, 155)
  arc A14 (-104.1961, 154.0194) -> (-105, 155) centre (-104, 155) ccw
  line L20 (-104.1961, 154.0194) -> (-104.8039, 150.9806)
  arc A15 (-104, 150) -> (-104.8039, 150.9806) centre (-105, 150) ccw
  line L21 (-104, 150) -> (-82.5, 150)
  circle A16 centre (-126.15, 162.5) radius 11.5
  dimension "d1101" = 23
  measures "d1101" diameter of A16
sketch "Sketch142" plane through (0, 0, -12.5) normal (0, 0, -1) x (1, 0, 0)
  line L0 (85, 175) -> (75, 175)
  line L1 (75, 175) -> (75, 150)
  line L2 (75, 150) -> (104, 150)
  arc A0 (104.8039, 150.9806) -> (104, 150) centre (105, 150) ccw
  line L3 (104.8039, 150.9806) -> (104.1961, 154.0194)
  arc A1 (105, 155) -> (104.1961, 154.0194) centre (104, 155) ccw
  line L4 (105, 155) -> (110, 155)
  arc A2 (110.8039, 154.0194) -> (110, 155) centre (111, 155) ccw
  line L5 (110.8039, 154.0194) -> (110.1961, 150.9806)
  arc A3 (111, 150) -> (110.1961, 150.9806) centre (110, 150) ccw
  line L6 (111, 150) -> (141.3, 150)
  arc A4 (142.1039, 150.9806) -> (141.3, 150) centre (142.3, 150) ccw
  line L7 (142.1039, 150.9806) -> (141.4961, 154.0194)
  arc A5 (142.3, 155) -> (141.4961, 154.0194) centre (141.3, 155) ccw
  line L8 (142.3, 155) -> (147.3, 155)
  arc A6 (148.1039, 154.0194) -> (147.3, 155) centre (148.3, 155) ccw
  line L9 (148.1039, 154.0194) -> (147.4961, 150.9806)
  arc A7 (148.3, 150) -> (147.4961, 150.9806) centre (147.3, 150) ccw
  line L10 (148.3, 150) -> (177.3, 150)
  line L11 (177.3, 150) -> (177.3, 175)
  line L12 (177.3, 175) -> (167.3, 175)
  line L13 (167.3, 175) -> (148.3, 175)
  arc A8 (147.4961, 174.0194) -> (148.3, 175) centre (147.3, 175) ccw
  line L14 (147.4961, 174.0194) -> (148.1039, 170.9806)
  arc A9 (147.3, 170) -> (148.1039, 170.9806) centre (148.3, 170) ccw
  line L15 (147.3, 170) -> (142.3, 170)
  arc A10 (141.4961, 170.9806) -> (142.3, 170) centre (141.3, 170) ccw
  line L16 (141.4961, 170.9806) -> (142.1039, 174.0194)
  arc A11 (141.3, 175) -> (142.1039, 174.0194) centre (142.3, 175) ccw
  line L17 (141.3, 175) -> (111, 175)
  arc A12 (110.1961, 174.0194) -> (111, 175) centre (110, 175) ccw
  line L18 (110.1961, 174.0194) -> (110.8039, 170.9806)
  arc A13 (110, 170) -> (110.8039, 170.9806) centre (111, 170) ccw
  line L19 (110, 170) -> (105, 170)
  arc A14 (104.1961, 170.9806) -> (105, 170) centre (104, 170) ccw
  line L20 (104.1961, 170.9806) -> (104.8039, 174.0194)
  arc A15 (104, 175) -> (104.8039, 174.0194) centre (105, 175) ccw
  line L21 (104, 175) -> (85, 175)
  circle A16 centre (126.15, 162.5) radius 7.5
  dimension "d1102" = 15
  measures "d1102" diameter of A16
hole "Hole39" at (126.15, -162.5, 27.5) direction (0, 0, -1) diameter 26 depth 26 tip angle 180 bodies 10
hole "Hole40" at (126.15, -162.5, -12.5) direction (0, 0, 1) diameter 13.9 depth 14 tip angle 180 countersink diameter 15 countersink angle 30 bodies 10
sketch "Sketch145" plane through (0, 0, 10) normal (0, 0, 1) x (-1, 0, 0)
sketch "Sketch146" plane through (0, 0, 0) normal (0, 0, 1) x (1, 0, 0)
  line L0 (90, -110) -> (120, -110)
  line L1 (120, -110) -> (120, -135)
  line L2 (120, -135) -> (90, -135)
  line L3 (90, -135) -> (90, -110)
  dimension "d1127" = 30
  dimension "d1128" = 25
  constraint horizontal L0
  constraint vertical L1
  constraint horizontal L2
  constraint vertical L3
  measures "d1127" distance of L0.start L0.end
  measures "d1128" distance of L0.end L1.end
extrude "Extrude185" add sketch "Sketch146" against normal blind 3 bodies 9
sketch "Sketch147" plane through (90, 0, 0) normal (-1, 0, 0) x (0, -1, 0)
  line L0 (135, 0) -> (148, 0)
  line L1 (148, 0) -> (148, 10)
  line L2 (148, 10) -> (97, 10)
  line L3 (97, 10) -> (97, 0)
  line L4 (97, 0) -> (110, 0)
  line L5 (110, 0) -> (110, -3)
  line L6 (110, -3) -> (135, -3)
  line L7 (135, -3) -> (135, 0)
  circle A0 centre (114, 0) radius 1.5
  circle A1 centre (123.2, 0) radius 1.5
  dimension "d1131" = 3
  dimension "d1132" = 3
  dimension "d1133" = 9.2
  measures "d1131" diameter of A0
  measures "d1132" diameter of A1
  measures "d1133" distance of A0.centre A1.centre
extrude "Extrude186" cut sketch "Sketch147" against normal blind 30 contours A0 | A1 bodies 9
sketch "Sketch148" plane through (0, 0, 0) normal (0, 0, 1) x (1, 0, 0)
  line L0 (-150, 250) -> (-162, 250)
  line L1 (-162, 250) -> (-162, 254.7)
  line L2 (-162, 254.7) -> (-150, 254.7)
  line L3 (-150, 254.7) -> (-150, 250)
  circle A0 centre (-157, 252.35) radius 1.5
  dimension "d1138" = 12
  dimension "d1139" = 4.7
  dimension "d1140" = 3
  dimension "d1141" = 2.35
  dimension "d1142" = 7
  constraint horizontal L0
  constraint vertical L1
  constraint horizontal L2
  constraint vertical L3
  measures "d1138" distance of L0.start L0.end
  measures "d1139" distance of L0.start L2.end
  measures "d1140" diameter of A0
  measures "d1141" distance of L0 A0.centre
  measures "d1142" distance of L3 A0.centre
sketch "Sketch149" plane through (0, 254.7, 0) normal (0, 1, 0) x (-1, 0, 0)
  line L0 (144, 0) -> (150, 0)
  line L1 (150, 5) -> (144, 5)
  line L2 (144, 5) -> (144, 0)
  line L3 (144, 5) -> (149, 5)
  line L4 (149, 5) -> (149, 0)
  line L5 (149, 0) -> (144, 0)
  line L6 (144, 0) -> (144, 5)
  line L7 (150, 0) -> (150, 5)
  constraint horizontal L3
  constraint vertical L4
  constraint horizontal L5
  constraint vertical L6
  constraint coincident L0 L4.end
  constraint coincident L1.end L2.start
sketch "Sketch150" plane through (0, 0, 5) normal (0, 0, 1) x (-1, 0, 0)
  line L0 (144, -254.7) -> (144, -280.7)
  line L1 (144, -280.7) -> (149, -280.7)
  line L2 (149, -280.7) -> (149, -254.7)
  line L3 (149, -280.7) -> (144, -280.7)
  line L4 (144, -280.7) -> (144, -275.7)
  line L5 (144, -275.7) -> (149, -275.7)
  line L6 (149, -275.7) -> (149, -280.7)
  line L7 (149, -254.7) -> (144, -254.7)
  dimension "d1149" = 5
  constraint horizontal L3
  constraint vertical L4
  constraint horizontal L5
  constraint vertical L6
  constraint coincident L1.end L2.start
  measures "d1149" distance of L1.end L5.end
sketch "Sketch151" plane through (-149, 0, 0) normal (-1, 0, 0) x (0, -1, 0)
  line L0 (-275.7, 5) -> (-275.7, 33.7)
  line L1 (-275.7, 33.7) -> (-280.7, 33.7)
  line L2 (-280.7, 33.7) -> (-280.7, 5)
  line L3 (-275.7, 33.7) -> (-281.5831, 33.7)
  line L4 (-281.5831, 33.7) -> (-281.5831, 29.2)
  line L5 (-281.5831, 29.2) -> (-275.7, 29.2)
  line L6 (-275.7, 29.2) -> (-275.7, 33.7)
  line L7 (-280.7, 5) -> (-275.7, 5)
  dimension "d1152" = 4.5
  constraint horizontal L3
  constraint vertical L4
  constraint horizontal L5
  constraint vertical L6
  constraint coincident L0.end L1.start
  measures "d1152" distance of L0.end L5.end
sketch "Sketch152" plane through (0, 275.7, 0) normal (0, -1, 0) x (1, 0, 0)
  line L0 (-149, 33.7) -> (-164, 33.7)
  line L1 (-164, 33.7) -> (-164, 29.2)
  line L2 (-164, 29.2) -> (-149, 29.2)
  circle A0 centre (-162, 31.2) radius 1.5
  circle A1 centre (-152.8, 31.2) radius 1.5
  line L3 (-149, 29.2) -> (-149, 33.7)
  dimension "d1155" = 3
  dimension "d1156" = 3
  dimension "d1157" = 9.2
  dimension "d1158" = 2
  dimension "d1159" = 2.5
  dimension "d1160" = 2.5
  measures "d1155" diameter of A0
  measures "d1156" diameter of A1
  measures "d1157" horizontal distance of A0.centre A1.centre
  measures "d1158" distance of L1 A0.centre
  measures "d1159" distance of L0 A1.centre
  measures "d1160" distance of L0 A0.centre
sketch "Sketch153" plane through (0, 0, 1.5) normal (0, 0, 1) x (-1, 0, 0)
  circle A0 centre (-126.15, 162.5) radius 6.95
  line L0 (-129.7207, 150) -> (-122.5793, 150)
  arc A1 (-122.5793, 150) -> (-122.5793, 175) centre (-126.15, 162.5) ccw
  line L1 (-122.5793, 175) -> (-129.7207, 175)
  arc A2 (-129.7207, 175) -> (-129.7207, 150) centre (-126.15, 162.5) ccw
  circle A3 centre (-126.15, 162.5) radius 6.95
  constraint concentric A0 A3
hole "Hole42" at (126.15, -162.5, 1.5) direction (0, 0, -1) diameter 13.9 depth 15 tip angle 180 countersink diameter 15 countersink angle 30 bodies 10
sketch "Sketch154" plane through (0, 174.8202, 0) normal (0, 1, 0) x (-1, 0, 0)
  line L0 (160, 17.5) -> (168, 17.5)
  line L1 (168, 17.5) -> (168, 15)
  line L2 (168, 15) -> (160, 15)
  line L3 (160, 15) -> (160, 0)
  line L4 (160, 0) -> (175, 0)
  line L5 (175, 0) -> (175, 120)
  line L6 (175, 120) -> (160, 120)
  line L7 (160, 120) -> (160, 17.5)
sketch "Sketch155" plane through (-160, 0, 0) normal (1, 0, 0) x (0, 1, 0)
  line L0 (113.6202, 15) -> (104.8202, 15)
  line L1 (104.8202, 15) -> (104.8202, 0)
  line L2 (104.8202, 0) -> (174.8202, 0)
  line L3 (174.8202, 0) -> (174.8202, 15)
  line L4 (174.8202, 15) -> (166.0202, 15)
  line L5 (166.0202, 15) -> (166.0202, 17.5)
  line L6 (166.0202, 17.5) -> (174.8202, 17.5)
  line L7 (174.8202, 17.5) -> (174.8202, 120)
  line L8 (174.8202, 120) -> (164.8202, 120)
  arc A0 (114.8202, 120) -> (164.8202, 120) centre (139.8202, 120) ccw
  line L9 (114.8202, 120) -> (104.8202, 120)
  line L10 (104.8202, 120) -> (104.8202, 17.5)
  line L11 (104.8202, 17.5) -> (113.6202, 17.5)
  line L12 (113.6202, 17.5) -> (113.6202, 15)
  circle A1 centre (139.8202, 20.75) radius 8.5
  line L13 (174.8202, 17.5) -> (172, 17.5)
  line L14 (172, 17.5) -> (172, 35)
  line L15 (172, 35) -> (174.8202, 35)
  line L16 (174.8202, 35) -> (174.8202, 17.5)
  line L17 (174.8202, 110) -> (167.8202, 110)
  line L18 (167.8202, 110) -> (167.8202, 107.5)
  line L19 (167.8202, 107.5) -> (174.8202, 107.5)
  line L20 (174.8202, 107.5) -> (174.8202, 110)
  line L21 (104.8202, 110) -> (111.8202, 110)
  line L22 (111.8202, 110) -> (111.8202, 107.5)
  line L23 (111.8202, 107.5) -> (104.8202, 107.5)
  line L24 (104.8202, 107.5) -> (104.8202, 110)
  dimension "d1190" = 17.5
  dimension "d1219" = 7
  dimension "d1220" = 2.5
  dimension "d1221" = 10
  dimension "d1222" = 7
  dimension "d1223" = 2.5
  dimension "d1224" = 10
  constraint horizontal L13
  constraint vertical L14
  constraint horizontal L15
  constraint vertical L16
  constraint coincident L6.end L7.start
  constraint horizontal L17
  constraint vertical L18
  constraint horizontal L19
  constraint vertical L20
  constraint coincident L7 L17.start
  constraint horizontal L21
  constraint vertical L22
  constraint horizontal L23
  constraint vertical L24
  constraint coincident L10 L21.start
  measures "d1190" distance of L13.end L14.end
  measures "d1219" distance of L17.start L17.end
  measures "d1220" distance of L17.start L19.end
  measures "d1221" distance of L8 L17
  measures "d1222" distance of L21.start L21.end
  measures "d1223" distance of L21.start L23.end
  measures "d1224" distance of L9 L21
extrude "Extrude198" add sketch "Sketch155" along normal blind 20 contours L6 L7 L13 L14 L15 L16 bodies 1
sketch "Sketch156" plane through (0, 172, 0) normal (0, -1, 0) x (1, 0, 0)
  line L0 (-160, 35) -> (-160, 17.5)
  line L1 (-160, 17.5) -> (-140, 17.5)
  line L2 (-140, 17.5) -> (-140, 35)
  line L3 (-140, 35) -> (-160, 35)
  circle A0 centre (-142, 30.7) radius 1.5
  circle A1 centre (-142, 21.5) radius 1.5
  dimension "d1184" = 3
  dimension "d1185" = 3
  dimension "d1186" = 9.2
  dimension "d1187" = 4
  dimension "d1188" = 2
  dimension "d1189" = 2
  measures "d1184" diameter of A0
  measures "d1185" diameter of A1
  measures "d1186" vertical distance of A0.centre A1.centre
  measures "d1187" distance of L1 A1.centre
  measures "d1188" distance of L2 A0.centre
  measures "d1189" distance of L2 A1.centre
extrude "Extrude199" cut sketch "Sketch156" against normal blind 7.162 contours A0 | A1 bodies 1